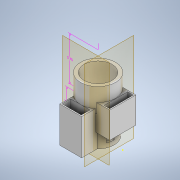
# Autodesk Inventor part: Housing
Saved by Autodesk Inventor 2021 (Build 250183000, 183)
## iProperties
Created: 2020-06-22
Part Number: Housing
Material: Generic
Document SubType Name: Modeling
Designer: Jaysonn
Density: 1 g/cm^3
Appearance: Default
Author: Jaysonn
## iProperties of the stored document _3DPrint.ipt
Created: 2020-06-24
Part Number: _3DPrint
Material: Generic
Document SubType Name: Modeling
Designer: Jaysonn
Density: 1 g/cm^3
Appearance: Default
Author: Jaysonn
Autodesk Inventor part; units mm, degrees
ref_plane "XZ Plane" through (0, 0, 0) normal (0, 1, 0) x (-1, 0, 0)
sketch "Sketch1" plane through (0, 0, 0) normal (0, 1, 0) x (-1, 0, 0)
  circle A0 centre (0, 0) radius 46.5
  dimension "d0" = 93
  constraints: 1 centre point, 1 coincident
  measures "d0" diameter of A0
extrude "Extrusion1" add sketch "Sketch1" along normal blind 90
sketch "Sketch2" plane through (0, 90, 0) normal (0, 1, 0) x (1, 0, 0)
  circle A0 centre (0, 0) radius 50.8
  dimension "d3" = 101.6
  constraints: 1 centre point, 1 coincident
  measures "d3" diameter of A0
extrude "Extrusion2" add sketch "Sketch2" along normal blind 146.05
sketch "Sketch4" plane through (0, 90, 0) normal (0, -1, 0) x (1, 0, 0)
  point P0 (0, 0)
sketch "Sketch5" plane through (0, 90, 0) normal (0, -1, 0) x (1, 0, 0)
  point P0 (0, 0)
sketch "Sketch6" plane through (0, 90, 0) normal (0, -1, 0) x (1, 0, 0)
  point P0 (0, 0)
fillet "Fillet1" radius 2 2 edges at (-50.8, 90, 0) (46.5, 90, 0)
ref_plane "Work Plane2" through (46.5, 0, 0) normal (1, 0, 0) x (0, 1, 0)
sketch "Sketch7" plane through (46.5, 0, 0) normal (1, 0, 0) x (0, 1, 0)
  line L0 (24.2179, 0) -> (12.6856, 0)
  line L1 (12.6856, 0) -> (12.6856, 18.4517)
  line L2 (12.6856, 18.4517) -> (24.2179, 18.4517)
  line L3 (24.2179, 18.4517) -> (24.2179, 0)
  point P0 (0, 0)
  constraints: 8 end point, 2 parallel, 1 horizontal, 1 perpendicular
extrude "Extrusion4" cut sketch "Sketch7" against normal blind 17.4625
sketch "Sketch12" plane through (0, 90, 0) normal (0, -1, 0) x (1, 0, 0)
  point P0 (0, 0)
sketch "Sketch13" plane through (0, 90, 0) normal (0, -1, 0) x (1, 0, 0)
  point P0 (0, 0)
sketch "Sketch14" plane through (0, 90, 0) normal (0, -1, 0) x (1, 0, 0)
  line L0 (65.7696, 29.9336) -> (57.3376, 29.9336)
  line L1 (57.3376, 29.9336) -> (57.3376, 7.1672)
  line L2 (57.3376, 7.1672) -> (65.7696, 7.1672)
  line L3 (65.7696, 7.1672) -> (65.7696, 29.9336)
  point P0 (0, 0)
  constraints: 8 end point, 2 parallel, 1 horizontal, 1 perpendicular
extrude "Extrusion8" cut sketch "Sketch14" against normal blind 141.605
ref_plane "Work Plane4" through (0, 0, 46.5) normal (0, 0, 1) x (1, 0, 0)
sketch "Sketch24" plane through (0, 0, 46.5) normal (0, 0, 1) x (1, 0, 0)
  point P0 (0, 0)
sketch "Sketch25" plane through (0, 0, 46.5) normal (0, 0, 1) x (1, 0, 0)
  line L0 (0, 0) -> (-31.75, 0)
  line L1 (-31.75, 0) -> (-31.75, 104.14)
  line L2 (-31.75, 104.14) -> (0, 104.14)
  line L3 (0, 104.14) -> (0, 0)
  line L4 (0, 0) -> (31.75, 0)
  line L5 (31.75, 0) -> (31.75, 104.14)
  line L6 (31.75, 104.14) -> (0, 104.14)
  line L7 (0, 104.14) -> (0, 0)
  dimension "d59" = 31.75
  dimension "d60" = 104.14
  dimension "d61" = 31.75
  dimension "d62" = 104.14
  constraints: 16 end point, 4 parallel, 2 horizontal, 2 perpendicular
  measures "d59" distance of L1.end L2.end
  measures "d60" distance of L0.end L1.end
  measures "d61" distance of L6.end L5.end
  measures "d62" distance of L5.end L4.end
extrude "Extrusion13" add sketch "Sketch25" along normal blind 33.02
sketch "Sketch26" plane through (0, 0, 79.52) normal (0, 0, 1) x (1, 0, 0)
  line L0 (-31.75, 104.14) -> (-31.75, 0) projected
  line L1 (0, 0) -> (31.75, 0) projected
  line L2 (-31.75, 104.14) -> (31.75, 104.14)
  line L3 (31.75, 104.14) -> (31.75, 0)
  line L4 (31.75, 0) -> (-31.75, 0)
  line L5 (-31.75, 0) -> (-31.75, 104.14)
  constraints: 8 end point, 2 parallel, 1 horizontal, 1 perpendicular
extrude "Extrusion14" add sketch "Sketch26" against normal blind 44.7675
sketch "Sketch27" plane through (0, 104.14, 0) normal (0, 1, 0) x (1, 0, 0)
  point P0 (0, 0)
sketch "Sketch28" plane through (0, 104.14, 0) normal (0, 1, 0) x (1, 0, 0)
  point P0 (0, 0)
sketch "Sketch29" plane through (0, 104.14, 0) normal (0, 1, 0) x (1, 0, 0)
  line L0 (-28.6575, -50.7647) -> (27.2225, -50.7647)
  line L1 (27.2225, -50.7647) -> (27.2225, -76.1647)
  line L2 (27.2225, -76.1647) -> (-28.6575, -76.1647)
  line L3 (-28.6575, -76.1647) -> (-28.6575, -50.7647)
  point P0 (0, 0)
  dimension "d67" = 55.88
  dimension "d68" = 25.4
  constraints: 8 end point, 2 parallel, 1 horizontal, 1 perpendicular
  measures "d67" distance of L1.end L2.end
  measures "d68" distance of L0.end L1.end
extrude "Extrusion15" cut sketch "Sketch29" against normal blind 98.1075
sketch "Sketch30" plane through (-31.75, 0, 79.52) normal (-1, 0, 0) x (0, 0, 1)
  line L0 (-0.5043, 102.352) -> (0, 76.957)
  line L1 (0, 0) -> (0, 104.14) projected
  line L2 (-24.2726, 76.475) -> (-9.0326, 76.475)
  line L3 (-9.0326, 76.475) -> (-9.0326, 38.375)
  line L4 (-9.0326, 38.375) -> (-24.2726, 38.375)
  line L5 (-24.2726, 38.375) -> (-24.2726, 76.475)
  point P0 (-79.52, 0)
  dimension "d71" = 25.4
  dimension "d72" = 15.24
  dimension "d73" = 38.1
  constraints: 10 end point, 2 parallel, 1 horizontal, 1 perpendicular, 1 point on line
  measures "d71" distance of L0.start L0.end
  measures "d72" distance of L3.end L4.end
  measures "d73" distance of L2.end L3.end
extrude "Extrusion16" cut sketch "Sketch30" against normal blind 46.355
ref_plane "Work Plane5" through (46.5, 0, 0) normal (1, 0, 0) x (0, 1, 0)
sketch "Sketch31" plane through (46.5, 0, 0) normal (1, 0, 0) x (0, 1, 0)
  line L0 (11.9436, 0) -> (43.6936, 0)
  line L1 (43.6936, 0) -> (119.8936, 0)
  line L2 (119.8936, 0) -> (119.8936, 38.1)
  line L3 (119.8936, 38.1) -> (43.6936, 38.1)
  line L4 (43.6936, 38.1) -> (43.6936, 0)
  line L5 (43.6936, 0) -> (119.8936, 0)
  line L6 (119.8936, 0) -> (119.8936, -38.1)
  line L7 (119.8936, -38.1) -> (43.6936, -38.1)
  line L8 (43.6936, -38.1) -> (43.6936, 0)
  point P0 (0, 0)
  dimension "d76" = 31.75
  dimension "d77" = 76.2
  dimension "d78" = 38.1
  dimension "d79" = 76.2
  dimension "d80" = 38.1
  constraints: 18 end point, 4 parallel, 3 horizontal, 2 perpendicular
  measures "d76" distance of L0.start L0.end
  measures "d77" distance of L3.end L2.end
  measures "d78" distance of L2.end L1.end
  measures "d79" distance of L6.end L7.end
  measures "d80" distance of L5.end L6.end
extrude "Extrusion17" add sketch "Sketch31" along normal blind 25.4
sketch "Sketch32" plane through (71.9, 0, 0) normal (1, 0, 0) x (0, 0, -1)
  point P0 (0, 0)
sketch "Sketch33" plane through (71.9, 0, 0) normal (1, 0, 0) x (0, 0, -1)
  line L0 (-20.4546, 119.8936) -> (-38.1, 119.8936) projected
  line L1 (0, 43.6936) -> (38.1, 43.6936) projected
  line L2 (-38.1, 119.8936) -> (38.1, 119.8936)
  line L3 (38.1, 119.8936) -> (38.1, 43.6936)
  line L4 (38.1, 43.6936) -> (-38.1, 43.6936)
  line L5 (-38.1, 43.6936) -> (-38.1, 119.8936)
  point P0 (0, 0)
  constraints: 8 end point, 2 parallel, 1 horizontal, 1 perpendicular
extrude "Extrusion18" add sketch "Sketch33" against normal blind 47.625
sketch "Sketch3" plane through (0, 236.05, 0) normal (0, 1, 0) x (1, 0, 0)
  circle A0 centre (0, 0) radius 40.64
  dimension "d6" = 81.28
  constraints: 1 centre point, 1 coincident
  measures "d6" diameter of A0
extrude "Extrusion3" cut sketch "Sketch3" against normal blind 228.6
sketch "Sketch34" plane through (33.601, 119.8936, 38.1) normal (0, 1, 0) x (1, 0, 0)
  line L0 (34.9589, 72.1697) -> (18.4489, 72.1697)
  line L1 (18.4489, 72.1697) -> (18.4489, 3.5897)
  line L2 (18.4489, 3.5897) -> (34.9589, 3.5897)
  line L3 (34.9589, 3.5897) -> (34.9589, 72.1697)
  point P0 (-33.601, 38.1)
  dimension "d85" = 16.51
  dimension "d86" = 68.58
  constraints: 8 end point, 2 parallel, 1 horizontal, 1 perpendicular
  measures "d85" distance of L2.end L1.end
  measures "d86" distance of L1.end L0.end
extrude "Extrusion19" cut sketch "Sketch34" against normal blind 71.4375
sketch "Sketch35" plane through (26.6578, 43.6936, -38.1) normal (0, -1, 0) x (1, 0, 0)
  point P0 (-26.6578, 38.1)
sketch "Sketch36" plane through (26.6578, 43.6936, -38.1) normal (0, -1, 0) x (1, 0, 0)
  line L0 (39.3784, 66.2811) -> (27.1807, 66.2811)
  line L1 (27.1807, 66.2811) -> (27.1807, 40.6237)
  line L2 (27.1807, 40.6237) -> (39.3784, 40.6237)
  line L3 (39.3784, 40.6237) -> (39.3784, 66.2811)
  point P0 (-26.6578, 38.1)
  constraints: 8 end point, 2 parallel, 1 horizontal, 1 perpendicular
extrude "Extrusion20" cut sketch "Sketch36" against normal blind 71.4375
sketch "Sketch37" plane through (0, 236.05, 0) normal (0, 1, 0) x (1, 0, 0)
  circle A0 centre (0, 0) radius 58.234
  constraints: 1 centre point, 1 coincident
extrude "Extrusion21" cut sketch "Sketch37" against normal blind 76.2
body "Solid1"
